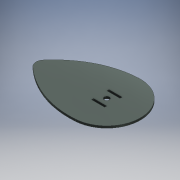
# Autodesk Inventor part: leva00
Saved by Autodesk Inventor 2016 (Build 200138000, 138)
## iProperties
Created: 2016-09-20
Part Number: leva00
Material: Madera (abedul)
Document SubType Name: Modeling
Designer: i95sa
Density: 0.55 g/cm^3
Appearance: Gris plomo - Pulido
Author: i95sa
Autodesk Inventor part; units mm, degrees
ref_plane "YZ Plane" through (0, 0, 0) normal (1, 0, 0) x (0, 1, 0)
ref_plane "XZ Plane" through (0, 0, 0) normal (0, 1, 0) x (-1, 0, 0)
ref_plane "XY Plane" through (0, 0, 0) normal (0, 0, 1) x (1, 0, 0)
sketch "Boceto1" plane through (0, 0, 0) normal (0, 0, 1) x (1, 0, 0)
  arc A0 (63.5094, 3.9957) -> (-63.5094, -3.9957) centre (0, 0) ccw
  arc A1 (-97.736, -6.149) -> (-127.0481, -7.9932) centre (-112.392, -7.0711) ccw
  line L0 (-131.2914, -8.2602) -> (-132.2134, 6.3959)
  line L1 (-3.2431, 63.5523) -> (-4.7799, 87.979)
  line L2 (-4.7799, 87.979) -> (-132.2134, 6.3959)
  line L3 (-132.2134, 6.3959) -> (-82.7429, 38.067)
  arc A2 (-3.2431, 63.5523) -> (-82.7429, 38.067) centre (5.0558, -99.0755) ccw
  arc A3 (-82.7429, 38.067) -> (-123.5703, 2.4523) centre (16.4017, -116.7978) ccw
  line L4 (4.8853, 0.3074) -> (63.5094, 3.9957)
  line L5 (-4.8853, -0.3074) -> (-131.2914, -8.2602)
  arc A4 (-63.5094, -3.9957) -> (63.5094, 3.9957) centre (0, 0) ccw
  arc A5 (-127.0481, -7.9932) -> (-97.736, -6.149) centre (-112.392, -7.0711) ccw
  line L6 (-131.2914, -8.2602) -> (-130.3693, -22.9162)
  line L7 (4.7477, -63.4576) -> (6.2845, -87.8843)
  line L8 (6.2845, -87.8843) -> (-130.3693, -22.9162)
  line L9 (-130.3693, -22.9162) -> (-77.3194, -48.1372)
  arc A6 (-77.3194, -48.1372) -> (4.7477, -63.4576) centre (-7.4015, 98.9279) ccw
  arc A7 (-122.2886, -17.9204) -> (-77.3194, -48.1372) centre (1.6337, 117.9325) ccw
  dimension "d0" = 127.27
  dimension "d6" = 29.37
  dimension "d7" = 14.685
  dimension "d8" = 24.475
  dimension "d9" = 58.74
  constraints: 20 end point, 20 point on circle, 8 centre point, 6 symmetric about line, 5 point on line, 4 tangent, 1 collinear, 4 other
  measures "d0" diameter of A0
  measures "d6" diameter of A1
  measures "d7" distance of L0.start L0.end
  measures "d8" distance of L1.start L1.end
  measures "d9" distance of L0.end L3.end
extrude "Extrusión2" add sketch "Boceto1" along normal blind 4 contours A4 A0 | A0 L5 A1 A3 A2 | A6 A7 A5 L5 A4 | L5 A1 | A5 L5
sketch "Boceto2" plane through (0, 0, 4) normal (0, 0, 1) x (1, 0, 0)
  line L0 (0, 0) -> (0, 12.5)
  line L1 (0, 12.5) -> (-12.5, 12.5)
  line L2 (-12.5, 12.5) -> (-12.5, 16.7)
  line L3 (-12.5, 16.7) -> (12.5, 16.7)
  line L4 (12.5, 16.7) -> (12.5, 12.5)
  line L5 (12.5, 12.5) -> (0, 12.5)
  line L6 (0, 0) -> (12.5, 0)
  line L7 (0, 0) -> (0, -12.5)
  line L8 (0, -12.5) -> (-12.5, -12.5)
  line L9 (-12.5, -12.5) -> (-12.5, -16.7)
  line L10 (-12.5, -16.7) -> (12.5, -16.7)
  line L11 (12.5, -16.7) -> (12.5, -12.5)
  line L12 (12.5, -12.5) -> (0, -12.5)
  circle A0 centre (0, 0) radius 5
  dimension "d24" = 12.5
  dimension "d25" = 12.5
  dimension "d26" = 4.2
  dimension "d27" = 25
  dimension "d28" = 10
  constraints: 26 end point, 5 perpendicular, 5 symmetric about line, 3 point on line, 1 centre point, 1 coincident, 1 parallel, 1 vertical
  measures "d24" distance of L0.start L0.end
  measures "d25" distance of L0.end L1.end
  measures "d26" distance of L1.end L2.end
  measures "d27" distance of L2.end L3.end
  measures "d28" diameter of A0
extrude "Extrusión3" cut sketch "Boceto2" against normal blind 4
